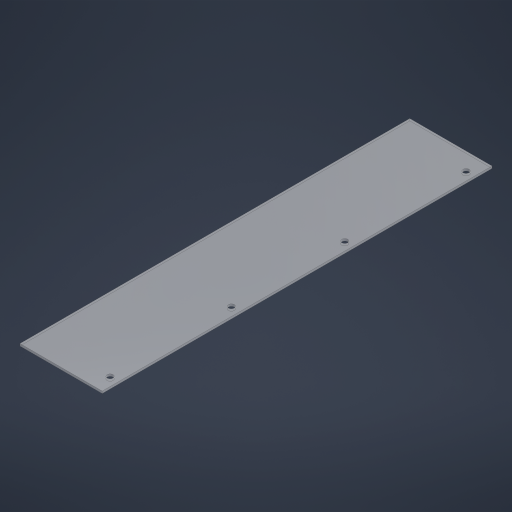
# Autodesk Inventor part: Bowling-Plastic
Saved by Autodesk Inventor 2024 (Build 280153000, 153)
## iProperties
Created: 2024-01-21
Part Number: Bowling-Plastic
Material: Polycarbonate, Clear
Document SubType Name: Sheet Metal
Designer: abhin
Density: 1.2 g/cm^3
Flat Pattern Width: 6.0325 cm
Flat Pattern Length: 28.575 cm
Flat Pattern Area: 172.379 cm^2
Sheet Metal Rule: Default
Sheet Metal Width: 2.375 in
Sheet Metal Length: 11.250 in
Sheet Metal Area: 26.719 in^2
Appearance: Polycarbonate - Clear
Author: abhin
Autodesk Inventor part; units mm, degrees
ref_plane "YZ Plane" through (0, 0, 0) normal (1, 0, 0) x (0, 1, 0)
ref_plane "XZ Plane" through (0, 0, 0) normal (0, 1, 0) x (-1, 0, 0)
ref_plane "XY Plane" through (0, 0, 0) normal (0, 0, 1) x (1, 0, 0)
sketch "Sketch1" plane through (0, 0, 0) normal (0, 1, 0) x (-1, 0, 0)
  line L0 (-30.1625, -142.875) -> (30.1625, -142.875)
  line L1 (30.1625, -142.875) -> (30.1625, 142.875)
  line L2 (30.1625, 142.875) -> (-30.1625, 142.875)
  line L3 (-30.1625, 142.875) -> (-30.1625, -142.875)
  line L4 (-30.1625, -142.875) -> (30.1625, 142.875) construction
  line L5 (30.1625, -142.875) -> (-30.1625, 142.875) construction
  point P0 (0, 0)
  dimension "d0" = 60.325
  dimension "d1" = 285.75
  constraints: 12 end point, 2 midpoint, 2 parallel, 1 horizontal, 1 perpendicular
  measures "d0" distance of L2.end L1.end
  measures "d1" distance of L1.end L0.end
extrude "Extrusion1" add sketch "Sketch1" along normal blind 1.5875
sketch "Sketch2" plane through (0, 1.5875, 0) normal (0, 1, 0) x (1, 0, 0)
  line L0 (30.055, -143.3465) -> (23.705, -143.3465)
  line L1 (23.705, -143.3465) -> (23.705, -130.6465)
  line L2 (23.705, -130.6465) -> (23.705, -41.7465)
  circle A0 centre (23.705, -130.6465) radius 2.1844
  circle A1 centre (23.705, -41.7465) radius 2.1844
  line L3 (30.1625, -142.875) -> (30.1625, 142.875) projected
  line L4 (30.1625, 142.875) -> (23.8125, 142.875)
  line L5 (23.8125, 142.875) -> (23.8125, 130.175)
  line L6 (23.8125, 130.175) -> (23.8125, 41.275)
  circle A2 centre (23.8125, 41.275) radius 2.1844
  circle A3 centre (23.8125, 130.175) radius 2.1844
  point P0 (0, 0)
  dimension "d4" = 6.35
  dimension "d5" = 12.7
  dimension "d6" = 88.9
  dimension "d7" = 4.3688
  dimension "d8" = 4.3688
  dimension "d9" = 6.35
  dimension "d10" = 12.7
  dimension "d11" = 88.9
  dimension "d12" = 4.3688
  dimension "d16" = 4.3688
  constraints: 12 end point, 4 centre point, 4 coincident, 2 horizontal, 2 perpendicular, 2 point on line
  measures "d4" distance of L0.start L0.end
  measures "d5" distance of L0.end L1.end
  measures "d6" distance of L1.end L2.end
  measures "d7" diameter of A0
  measures "d8" diameter of A1
  measures "d9" distance of L3.end L4.end
  measures "d10" distance of L4.end L5.end
  measures "d11" distance of L5.end L6.end
  measures "d12" diameter of A2
  measures "d16" diameter of A3
extrude "Extrusion2" cut sketch "Sketch2" against normal blind 1.5875
equation "\"BendRadius\" = Thickness"
equation "\"BendReliefWidth\" = Thickness"
equation "\"BendReliefDepth\" = 0.5 * Thickness"
equation "\"CornerReliefSize\" = 4 * Thickness"
equation "\"MinimumRemnant\" = 2 * Thickness"
equation "\"TransitionRadius\" = BendRadius"
equation "\"JacobiRadiusSize\" = BendRadius"
equation "\"GapSize\" = Thickness"
equation "\"Thickness\" = 1.5875"
body "Solid1"
